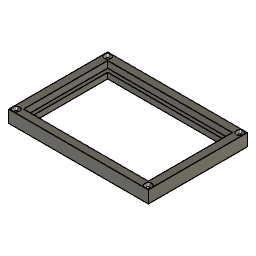
relayboxtop (1) (Autodesk Fusion 360 design; units mm, degrees)
part number: 2025-12-20-15-07-03-046
Autodesk Fusion 360 part; units mm, degrees
sketch "Sketch1" plane through (0, 0, 0) normal (0, 0, 1) x (1, 0, 0)
  line L0 (39.5, 28) -> (-39.5, 28)
  line L1 (-39.5, 28) -> (-39.5, -28)
  line L2 (-39.5, -28) -> (39.5, -28)
  line L3 (39.5, -28) -> (39.5, 28)
  line L4 (39.5, 28) -> (-39.5, -28) construction
  line L5 (-39.5, 28) -> (39.5, -28) construction
  dimension "d1" = 79
  dimension "d2" = 56
  constraint horizontal L0
  constraint perpendicular L0 L1
  constraint parallel L0 L2
  constraint parallel L1 L3
  constraint coincident L4 origin
  constraint coincident L5 origin
  measures "d1" distance of L1.end L2.end
  measures "d2" distance of L0.end L1.end
extrude "Extrude1" add sketch "Sketch1" along normal blind 7
sketch "Sketch2" plane through (0, 0, 7) normal (0, 0, 1) x (-1, 0, 0)
  line L0 (-39.5, 28) -> (-39.5, -28)
  line L1 (-39.5, -28) -> (39.5, -28)
  line L2 (39.5, -28) -> (39.5, 28)
  line L3 (39.5, 28) -> (-39.5, 28)
  line L4 (-35.25, -23.75) -> (35.25, -23.75)
  line L5 (35.25, -23.75) -> (35.25, 23.75)
  line L6 (35.25, 23.75) -> (-35.25, 23.75)
  line L7 (-35.25, 23.75) -> (-35.25, -23.75)
  line L8 (-35.25, -23.75) -> (35.25, 23.75) construction
  line L9 (35.25, -23.75) -> (-35.25, 23.75) construction
  dimension "d5" = 70.5
  dimension "d6" = 47.5
  constraint horizontal L4
  constraint perpendicular L4 L5
  constraint parallel L4 L6
  constraint parallel L5 L7
  constraint coincident L8 origin
  constraint coincident L9 origin
  measures "d5" distance of L5.end L6.end
  measures "d6" distance of L4.end L5.end
extrude "Extrude2" cut sketch "Sketch2" against normal blind 3.75 contours L4 L5 L6 L7
sketch "Sketch3" plane through (0, 0, 3.25) normal (0, 0, 1) x (-1, 0, 0)
  line L0 (-35.25, 23.75) -> (-35.25, -23.75)
  line L1 (-35.25, -23.75) -> (35.25, -23.75)
  line L2 (35.25, -23.75) -> (35.25, 23.75)
  line L3 (35.25, 23.75) -> (-35.25, 23.75)
  line L4 (33.25, 21.75) -> (-33.25, 21.75)
  line L5 (-33.25, 21.75) -> (-33.25, -21.75)
  line L6 (-33.25, -21.75) -> (33.25, -21.75)
  line L7 (33.25, -21.75) -> (33.25, 21.75)
  line L8 (33.25, 21.75) -> (-33.25, -21.75) construction
  line L9 (-33.25, 21.75) -> (33.25, -21.75) construction
  dimension "d9" = 66.5
  dimension "d10" = 43.5
  constraint horizontal L4
  constraint perpendicular L4 L5
  constraint parallel L4 L6
  constraint parallel L5 L7
  constraint coincident L8 origin
  constraint coincident L9 origin
  measures "d9" distance of L5.end L6.end
  measures "d10" distance of L4.end L5.end
extrude "Extrude3" cut sketch "Sketch3" against normal blind 3.25 contours L4 L5 L6 L7
sketch "Sketch4" plane through (0, 0, 7) normal (0, 0, 1) x (-1, 0, 0)
  line L0 (35.25, -23.75) -> (-35.25, -23.75)
  line L1 (-35.25, -23.75) -> (-35.25, 23.75)
  line L2 (-35.25, 23.75) -> (35.25, 23.75)
  line L3 (35.25, 23.75) -> (35.25, -23.75)
  line L4 (-39.5, 28) -> (-39.5, -28)
  line L5 (-39.5, -28) -> (39.5, -28)
  line L6 (39.5, -28) -> (39.5, 28)
  line L7 (39.5, 28) -> (-39.5, 28)
  circle A0 centre (37.375, -25.875) radius 2
  dimension "d13" = 4
  dimension "d14" = 2.125
  dimension "d15" = 2.125
  measures "d13" diameter of A0
  measures "d14" distance of L5 A0.centre
  measures "d15" distance of L6 A0.centre
sketch "Sketch5" plane through (0, 0, 7) normal (0, 0, 1) x (-1, 0, 0)
  line L0 (35.25, -23.75) -> (-35.25, -23.75)
  line L1 (-35.25, -23.75) -> (-35.25, 23.75)
  line L2 (-35.25, 23.75) -> (35.25, 23.75)
  line L3 (35.25, 23.75) -> (35.25, -23.75)
  line L4 (-39.5, 28) -> (-39.5, -28)
  line L5 (-39.5, -28) -> (39.5, -28)
  line L6 (39.5, -28) -> (39.5, 28)
  line L7 (39.5, 28) -> (-39.5, 28)
  circle A0 centre (-37.375, -25.875) radius 2
  circle A1 centre (-37.375, 25.875) radius 2
  circle A2 centre (37.375, 25.875) radius 2
  dimension "d23" = 4
  dimension "d24" = 2.125
  dimension "d25" = 2.125
  dimension "d26" = 4
  dimension "d27" = 2.125
  dimension "d28" = 2.125
  dimension "d29" = 4
  dimension "d30" = 2.125
  dimension "d31" = 2.125
  measures "d23" diameter of A0
  measures "d24" distance of L5 A0.centre
  measures "d25" distance of L4 A0.centre
  measures "d26" diameter of A1
  measures "d27" distance of L4 A1.centre
  measures "d28" distance of L7 A1.centre
  measures "d29" diameter of A2
  measures "d30" distance of L7 A2.centre
  measures "d31" distance of L6 A2.centre
hole "Hole2" at (37.375, 25.875, 7) at (37.375, -25.875, 7) at (-37.375, -25.875, 7) direction (0, 0, -1) diameter 1.6256 depth 7.0104 tip angle 180 countersink diameter 3.9878 countersink angle 90
thread "Thread2" "ISO Metric profile 2.0 M2x0.4 M2x0.4 6H" thread offset 0 thread depth 5.9436
sketch "Sketch6" plane through (0, 0, 7) normal (0, 0, 1) x (-1, 0, 0)
  circle A0 centre (-37.375, 25.875) radius 1.9939
  circle A1 centre (-37.375, -25.875) radius 1.9939
  circle A2 centre (37.375, 25.875) radius 1.9939
  line L0 (35.25, -23.75) -> (-35.25, -23.75)
  line L1 (-35.25, -23.75) -> (-35.25, 23.75)
  line L2 (-35.25, 23.75) -> (35.25, 23.75)
  line L3 (35.25, 23.75) -> (35.25, -23.75)
  line L4 (-39.5, 28) -> (-39.5, -28)
  line L5 (-39.5, -28) -> (39.5, -28)
  line L6 (39.5, -28) -> (39.5, 28)
  line L7 (39.5, 28) -> (-39.5, 28)
  circle A3 centre (37.375, -25.875) radius 2
  dimension "d39" = 4
  dimension "d40" = 2.125
  dimension "d41" = 2.125
  measures "d39" diameter of A3
  measures "d40" distance of L5 A3.centre
  measures "d41" distance of L6 A3.centre
hole "Hole3" at (-37.375, 25.875, 7) direction (0, 0, -1) diameter 1.6256 depth 7.0104 tip angle 180 countersink diameter 3.9878 countersink angle 90
thread "Thread3" "ISO Metric profile 2.0 M2x0.4 M2x0.4 6H" thread offset 0 thread depth 5.9436
sketch "Sketch7" plane through (0, 0, 3.25) normal (0, 0, 1) x (-1, 0, 0)
  line L0 (-33.25, 21.75) -> (33.25, 21.75)
  line L1 (33.25, 21.75) -> (33.25, -21.75)
  line L2 (33.25, -21.75) -> (-33.25, -21.75)
  line L3 (-33.25, -21.75) -> (-33.25, 21.75)
  line L4 (-35.25, 23.75) -> (-35.25, -23.75)
  line L5 (-35.25, -23.75) -> (35.25, -23.75)
  line L6 (35.25, -23.75) -> (35.25, 23.75)
  line L7 (35.25, 23.75) -> (-35.25, 23.75)
sketch "Sketch8" plane through (35.25, 0, 0) normal (-1, 0, 0) x (0, -1, 0)
  line L0 (23.75, 7) -> (-23.75, 7)
  line L1 (-23.75, 7) -> (-23.75, 3.25)
  line L2 (-23.75, 3.25) -> (23.75, 3.25)
  line L3 (23.75, 3.25) -> (23.75, 7)
